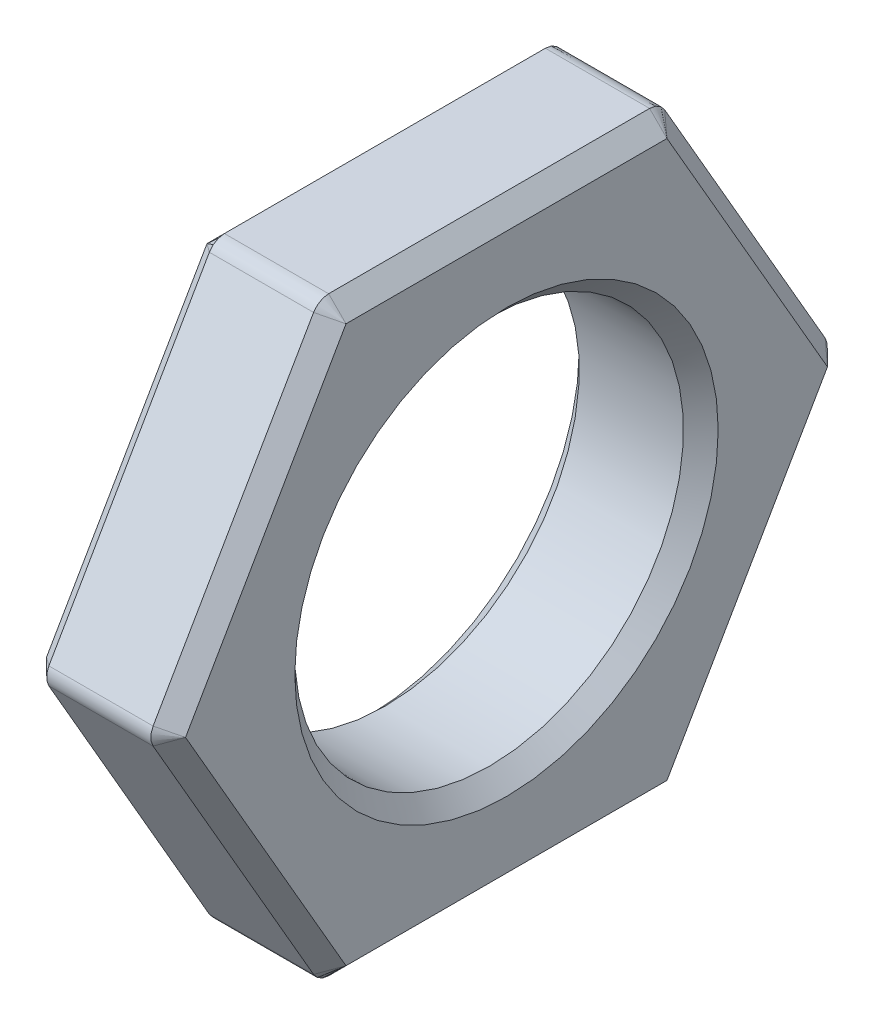
# Autodesk Inventor part: tuerca
Saved by Autodesk Inventor 2021 (Build 250183000, 183)
## iProperties
Created: 2021-04-24
Part Number: tuerca
Material: Genérico
Document SubType Name: Modeling
Designer: j2seb
Density: 1 g/cm^3
Appearance: Valor por defecto
Author: j2seb
Autodesk Inventor part; units mm, degrees
ref_plane "YZ Plane" through (0, 0, 0) normal (1, 0, 0) x (0, 1, 0)
ref_plane "XZ Plane" through (0, 0, 0) normal (0, 1, 0) x (-1, 0, 0)
ref_plane "XY Plane" through (0, 0, 0) normal (0, 0, 1) x (1, 0, 0)
sketch "Boceto1" plane through (0, 0, 0) normal (1, 0, 0) x (0, 1, 0)
  line L0 (17, 9.815) -> (17, -9.815)
  line L1 (17, 9.815) -> (0, 0) construction
  line L2 (0, 0) -> (17, -9.815) construction
  line L3 (0, 0) -> (17, 9.815) construction
  line L4 (0, 19.6299) -> (17, 9.815)
  line L5 (0, 19.6299) -> (0, 0) construction
  line L6 (0, 0) -> (0, 19.6299) construction
  line L7 (-17, 9.815) -> (0, 19.6299)
  line L8 (-17, 9.815) -> (0, 0) construction
  line L9 (0, 0) -> (-17, 9.815) construction
  line L10 (-17, -9.815) -> (-17, 9.815)
  line L11 (-17, -9.815) -> (0, 0) construction
  line L12 (0, 0) -> (-17, -9.815) construction
  line L13 (0, -19.6299) -> (-17, -9.815)
  line L14 (0, -19.6299) -> (0, 0) construction
  line L15 (0, 0) -> (0, -19.6299) construction
  line L16 (17, -9.815) -> (0, -19.6299)
  line L17 (17, -9.815) -> (0, 0) construction
  point P0 (17, 0)
  point P1 (8.5, 14.7224)
  point P2 (-8.5, 14.7224)
  point P3 (-17, 0)
  point P4 (-8.5, -14.7224)
  point P5 (8.5, -14.7224)
  point P6 (17, 9.815)
  point P7 (0, 19.6299)
  point P8 (-17, 9.815)
  point P9 (-17, -9.815)
  point P10 (0, -19.6299)
  point P11 (17, -9.815)
  dimension "d1" = 60
  dimension "d2" = 17
  dimension "d5" = 360
  constraints: 36 end point, 3 coincident, 1 horizontal alignment, 1 midpoint, 1 vertical, 41 other
  measures "d1" angle of L2 L1
  measures "d2" distance from line of L1.end L0
extrude "Extrusión1" add sketch "Boceto1" along normal blind 8
hole "Agujero1" at (0, 0, 0) direction (1, 0, 0) diameter 22.3762 end through all thread size "M24x1.5" class "6H" standard "ISO Metric profile"
fillet "Empalme1" radius 1 6 edges at (4, 17, -9.815) (4, 0, -19.6299) (4, -17, -9.815) (4, 17, 9.815) (4, 0, 19.6299) (4, -17, 9.815)
chamfer "Chaflán1" distance 1 angle 45 24 edges at (8, 17, 0) (8, 16.866, 9.7376) (8, 8.5, 14.7224) (8, 0, 19.4752) (8, -8.5, 14.7224) (8, -16.866, 9.7376) (8, -17, 0) (8, -16.866, -9.7376) (8, -8.5, -14.7224) (8, 0, -19.4752) (8, 8.5, -14.7224) (8, 16.866, -9.7376) (0, 17, 0) (0, 16.866, 9.7376) (0, 8.5, 14.7224) (0, 0, 19.4752) (0, -8.5, 14.7224) (0, -16.866, 9.7376) (0, -17, 0) (0, -16.866, -9.7376) (0, -8.5, -14.7224) (0, 0, -19.4752) (0, 8.5, -14.7224) (0, 16.866, -9.7376)
chamfer "Chaflán2" distance 1 angle 45 2 edges at (0, 0, -11.1881) (8, 0, -11.1881)
